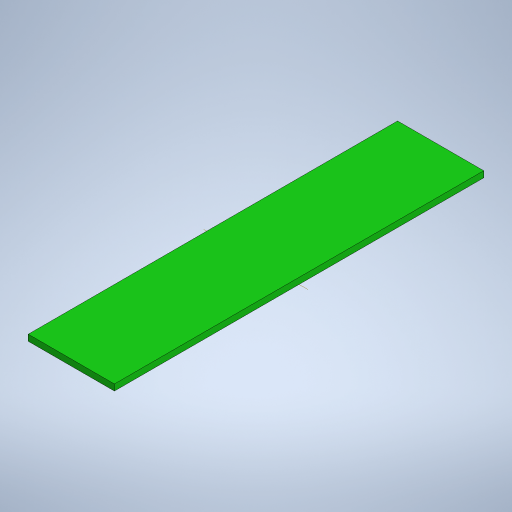
# Autodesk Inventor part: MCU_PCB
Saved by Autodesk Inventor 2024 (Build 280153000, 153)
## iProperties
Created: 2025-02-15
Part Number: MCU_PCB
Material: Generic
Document SubType Name: Modeling
Designer: XxPan
Density: 1 g/cm^3
Appearance: Default
Author: XxPan
Autodesk Inventor part; units mm, degrees
ref_plane "YZ Plane" through (0, 0, 0) normal (1, 0, 0) x (0, 1, 0)
ref_plane "XZ Plane" through (0, 0, 0) normal (0, 1, 0) x (-1, 0, 0)
ref_plane "XY Plane" through (0, 0, 0) normal (0, 0, 1) x (1, 0, 0)
sketch "Sketch1" plane through (0, 0, 0) normal (0, 1, 0) x (-1, 0, 0)
  line L0 (7, 30) -> (-7, 30)
  line L1 (-7, 30) -> (-7, -30)
  line L2 (-7, -30) -> (7, -30)
  line L3 (7, -30) -> (7, 30)
  line L4 (9.8, 0) -> (-9.8, 0) construction
  line L5 (0, -42) -> (0, 42) construction
  point P0 (0, 0)
  point P1 (7, 0)
  point P2 (0, 30)
  dimension "d0" = 14
  dimension "d1" = 60
  constraints: 8 end point, 2 midpoint, 2 parallel, 2 point on line, 1 horizontal, 1 perpendicular
  measures "d0" distance of L2.end L1.end
  measures "d1" distance of L2.end L0.start
extrude "Extrusion1" add sketch "Sketch1" along normal blind 1
body "Solid1"
